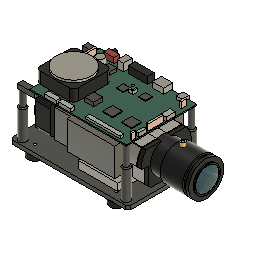
Projector v8 (Autodesk Fusion 360 design; units mm, degrees)
Autodesk Fusion 360 part; units mm, degrees
note: some values were not read from the file. Set by a fixed rule: which sketch regions a step uses.
sketch "Sketch1" plane through (0, 0, 0) normal (0, 0, 1) x (1, 0, 0)
  line L0 (0, 0) -> (155.5, 0)
  line L1 (155.5, 0) -> (155.5, 100)
  line L2 (155.5, 100) -> (0, 100)
  line L3 (0, 100) -> (0, 0)
  dimension "d1" = 155.5
  dimension "d2" = 100
  constraint horizontal L0
  constraint vertical L1
  constraint horizontal L2
  constraint vertical L3
  constraint coincident L0.start L3.end
  measures "d1" distance of L0.start L0.end
  measures "d2" distance of L0.start L2.end
extrude "Extrude1" add sketch "Sketch1" along normal blind 5 makes body 1
sketch "Sketch3" plane through (0, 0, 0) normal (0, 0, -1) x (1, 0, 0)
  line L0 (0, 0) -> (0, -100)
  line L1 (0, -100) -> (155.5, -100)
  line L2 (155.5, -100) -> (155.5, 0)
  line L3 (155.5, 0) -> (0, 0)
  line L4 (9.75, -7.15) -> (145.75, -7.15)
  line L5 (145.75, -7.15) -> (145.75, -92.85)
  line L6 (145.75, -92.85) -> (9.75, -92.85)
  line L7 (9.75, -92.85) -> (9.75, -7.15)
  line L8 (0, -50) -> (155.5, -50) construction
  line L9 (77.75, 0) -> (77.75, -100) construction
  line L10 (23, -9.75) -> (130.5, -9.75)
  line L11 (130.5, -9.75) -> (130.5, -90.25)
  line L12 (130.5, -90.25) -> (23, -90.25)
  line L13 (23, -90.25) -> (23, -9.75)
  dimension "d5" = 136
  dimension "d6" = 85.7
  dimension "d13" = 107.5
  dimension "d14" = 80.5
  dimension "d15" = 25
  dimension "d16" = 23
  constraint horizontal L4
  constraint vertical L5
  constraint horizontal L6
  constraint vertical L7
  constraint midpoint L0 L8.start
  constraint midpoint L2 L8.end
  constraint midpoint L3 L9.start
  constraint midpoint L1 L9.end
  constraint symmetric L4 L6 L8
  constraint symmetric L5 L7 L9
  constraint horizontal L10
  constraint vertical L11
  constraint horizontal L12
  constraint vertical L13
  constraint symmetric L8 L10 L12
  measures "d5" distance of L4.start L4.end
  measures "d6" distance of L4.start L6.end
  measures "d13" distance of L10.start L10.end
  measures "d14" distance of L10.end L11.end
  measures "d15" distance of L2 L11
  measures "d16" distance of L0 L13
hole "Hole1" at (9.75, 7.15, 0) at (145.75, 7.15, 0) at (145.75, 92.85, 0) at (9.75, 92.85, 0) direction (0, 0, 1) diameter 3 depth 5 tip angle 180 counterbore diameter 8 counterbore depth 3.5 bodies 1
chamfer "Chamfer1" distance 3.5 angle 45 4 edges at (0, 0, 2.5) (155.5, 0, 2.5) (0, 100, 2.5) (155.5, 100, 2.5) on bodies 1
hole "Hole2" at (23, 9.75, 0) at (130.5, 9.75, 0) at (130.5, 90.25, 0) at (23, 90.25, 0) direction (0, 0, 1) diameter 3.332 depth 5 tip angle 180 bodies 1
thread "Thread1" "ISO Metric profile 4.0 M4x0.7 6H"
sketch "Sketch4" plane through (0, 0, 0) normal (0, 0, 1) x (1, 0, 0) in component "Rubber Leg"
  circle A0 centre (0, 0) radius 10
  dimension "d20" = 20
  constraint coincident A0.centre origin
  measures "d20" diameter of A0
extrude "Extrude2" add sketch "Sketch4" along normal blind 8 separate body makes body 2 in component "Rubber Leg"
hole "Hole3" at (0, 0, 8) direction (0, 0, -1) diameter 4 depth 8 tip angle 180 counterbore diameter 8 counterbore depth 5 bodies 2 in component "Rubber Leg"
chamfer "Chamfer1'" distance 1 distance2 8 1 edges at (-9.3233, -3.6162, 8) measured on face at (7.959, -0.5964, 8) on bodies 2 in component "Rubber Leg"
pattern_linear "ఁ4" [suppressed]
sketch "Sketch2" plane through (0, 0, 0) normal (0, 0, 1) x (1, 0, 0) in component "Short Pole"
  circle A0 centre (0, 0) radius 5
  dimension "d38" = 10
  constraint coincident A0.centre origin
  measures "d38" diameter of A0
extrude "Extrude1'" add sketch "Sketch2" along normal blind 39 separate body makes body 3 in component "Short Pole"
sketch "Sketch3 (2)" plane through (0, 0, 39) normal (0, 0, 1) x (-1, 0, 0) in component "Short Pole"
  circle A0 centre (0, 0) radius 5
  circle A1 centre (0, 0) radius 3.5
  dimension "d41" = 7
  constraint coincident A0.centre A1.centre
  measures "d41" diameter of A1
extrude "Extrude2'" add sketch "Sketch3 (2)" along normal blind 19 contours A1 bodies 3 in component "Short Pole"
chamfer "Chamfer1''" distance 1.5 angle 45 1 edges at (-4.6616, -1.8081, 39) on bodies 3 in component "Short Pole"
sketch "Sketch2 (2)" plane through (0, 0, 0) normal (0, 0, 1) x (1, 0, 0) in component "Short Pole (1)"
  circle A0 centre (0, 0) radius 5
  dimension "d38_1" = 10
  constraint coincident A0.centre origin
  measures "d38_1" diameter of A0
extrude "Extrude1''" add sketch "Sketch2 (2)" along normal blind 39 separate body makes body 4 in component "Short Pole (1)"
sketch "Sketch3 (3)" plane through (0, 0, 39) normal (0, 0, 1) x (-1, 0, 0) in component "Short Pole (1)"
  circle A0 centre (0, 0) radius 5
  circle A1 centre (0, 0) radius 3.5
  dimension "d41_1" = 7
  constraint coincident A0.centre A1.centre
  measures "d41_1" diameter of A1
extrude "Extrude2''" add sketch "Sketch3 (3)" along normal blind 19 contours A1 bodies 4 in component "Short Pole (1)"
chamfer "Chamfer1'''" distance 1.5 angle 45 1 edges at (-4.6616, -1.8081, 39) on bodies 4 in component "Short Pole (1)"
sketch "Sketch2 (3)" plane through (0, 0, 0) normal (0, 0, 1) x (1, 0, 0) in component "Tall Pole"
  circle A0 centre (0, 0) radius 5
  dimension "d38_2" = 10
  constraint coincident A0.centre origin
  measures "d38_2" diameter of A0
extrude "Extrude1'''" add sketch "Sketch2 (3)" along normal blind 39 separate body makes body 5 in component "Tall Pole"
sketch "Sketch3 (4)" plane through (0, 0, 39) normal (0, 0, 1) x (-1, 0, 0) in component "Tall Pole"
  circle A0 centre (0, 0) radius 5
  circle A1 centre (0, 0) radius 3.5
  dimension "d41_2" = 7
  constraint coincident A0.centre A1.centre
  measures "d41_2" diameter of A1
extrude "Extrude2'''" add sketch "Sketch3 (4)" along normal blind 25 contours A1 bodies 5 in component "Tall Pole"
chamfer "Chamfer1''''" distance 1.5 angle 45 1 edges at (-4.6616, -1.8081, 39) on bodies 5 in component "Tall Pole"
sketch "Sketch2 (4)" plane through (0, 0, 0) normal (0, 0, 1) x (1, 0, 0) in component "Tall Pole (1)"
  circle A0 centre (0, 0) radius 5
  dimension "d38_1_1" = 10
  constraint coincident A0.centre origin
  measures "d38_1_1" diameter of A0
extrude "Extrude1''''" add sketch "Sketch2 (4)" along normal blind 39 separate body makes body 6 in component "Tall Pole (1)"
sketch "Sketch3 (5)" plane through (0, 0, 39) normal (0, 0, 1) x (-1, 0, 0) in component "Tall Pole (1)"
  circle A0 centre (0, 0) radius 5
  circle A1 centre (0, 0) radius 3.5
  dimension "d41_1_1" = 7
  constraint coincident A0.centre A1.centre
  measures "d41_1_1" diameter of A1
extrude "Extrude2''''" add sketch "Sketch3 (5)" along normal blind 25 contours A1 bodies 6 in component "Tall Pole (1)"
chamfer "Chamfer1'''''" distance 1.5 angle 45 1 edges at (-4.6616, -1.8081, 39) on bodies 6 in component "Tall Pole (1)"
sketch "Sketch6" plane through (-9.75, -7.15, 58) normal (0, 0, 1) x (-1, 0, 0) in component "Short Pole"
  circle A0 centre (-9.75, -7.15) radius 3.5
  line L0 (-6.25, -3.65) -> (-29.25, -3.65)
  line L1 (-29.25, -3.65) -> (-29.25, -10.65)
  line L2 (-29.25, -10.65) -> (-6.25, -10.65)
  line L3 (-6.25, -10.65) -> (-6.25, -3.65)
  dimension "d53" = 23
  dimension "d54" = 7
  constraint horizontal L0
  constraint vertical L1
  constraint horizontal L2
  constraint vertical L3
  constraint tangent A0 L2
  constraint tangent A0 L3
  measures "d53" distance of L0.start L0.end
  measures "d54" distance of L0.start L2.end
extrude "Extrude3" add sketch "Sketch6" along normal blind 6 separate body makes body 7 in component "Short Pole"
sketch "Sketch4 (2)" plane through (0, 0, 58) normal (0, 0, 1) x (-1, 0, 0) in component "Short Pole (1)"
  circle A0 centre (0, 0) radius 3.5
  line L0 (3.5, -3.5) -> (-19.5, -3.5)
  line L1 (-19.5, -3.5) -> (-19.5, 3.5)
  line L2 (-19.5, 3.5) -> (3.5, 3.5)
  line L3 (3.5, 3.5) -> (3.5, -3.5)
  dimension "d57" = 23
  dimension "d58" = 7
  constraint horizontal L0
  constraint vertical L1
  constraint horizontal L2
  constraint vertical L3
  constraint tangent A0 L0
  constraint tangent A0 L3
  measures "d57" distance of L0.start L0.end
  measures "d58" distance of L0.start L2.end
extrude "Extrude3'" add sketch "Sketch4 (2)" along normal blind 6 bodies 4 in component "Short Pole (1)"
ref_plane "WorkPlane1" through (77.75, 50, 69) normal (0, 0, 1) x (1, 0, 0)
sketch "Sketch7" plane through (77.75, 50, 69) normal (0, 0, 1) x (1, 0, 0)
  line L0 (-71.5, 39.35) -> (-48.5, 39.35)
  line L1 (-48.5, 39.35) -> (-48.5, 46.35)
  line L2 (-48.5, 46.35) -> (-71.5, 46.35)
  line L3 (-71.5, 46.35) -> (-71.5, 39.35)
  line L4 (-71.5, -39.35) -> (-71.5, -46.35)
  line L5 (-71.5, -46.35) -> (-48.5, -46.35)
  line L6 (-48.5, -46.35) -> (-48.5, -39.35)
  line L7 (-48.5, -39.35) -> (-71.5, -39.35)
  circle A0 centre (68, 42.85) radius 3.5
  circle A1 centre (68, -42.85) radius 3.5
  line L8 (-55.5, 46.35) -> (71.5, 46.35)
  line L9 (71.5, 46.35) -> (71.5, -46.35)
  line L10 (71.5, -46.35) -> (-55.5, -46.35)
  line L11 (-55.5, -46.35) -> (-55.5, 46.35)
  dimension "d62" = 7
  constraint horizontal L8
  constraint vertical L9
  constraint horizontal L10
  constraint vertical L11
  constraint tangent A0 L8
  constraint tangent A1 L10
  constraint tangent A1 L9
  measures "d62" distance of L1 L11
extrude "Extrude3''" add sketch "Sketch7" along normal blind 1.5 separate body contours L0 L1 L2 L8 L11 | L0 L1 L6 L7 A0 A1 L8 L9 L10 L11 | L5 L6 L7 L10 L11 | A0 L8 L9 | A0 | A1 | A1 L9 L10 makes body 8
ref_plane "WorkPlane2" through (85.75, 50, 79) normal (0, 0, 1) x (1, 0, 0)
sketch "Sketch9" plane through (85.75, 50, 79) normal (0, 0, 1) x (1, 0, 0)
  line L0 (-63.5, -46.35) -> (63.5, -46.35)
  line L1 (63.5, -46.35) -> (63.5, 46.35)
  line L2 (63.5, 46.35) -> (-63.5, 46.35)
  line L3 (-63.5, 46.35) -> (-63.5, -46.35)
  line L4 (-59.5, -42.35) -> (-9.5, -42.35)
  line L5 (-9.5, -42.35) -> (-9.5, 7.65)
  line L6 (-9.5, 7.65) -> (-59.5, 7.65)
  line L7 (-59.5, 7.65) -> (-59.5, -42.35)
  dimension "d68" = 50
  dimension "d69" = 50
  dimension "d70" = 4
  dimension "d71" = 4
  constraint horizontal L4
  constraint vertical L5
  constraint horizontal L6
  constraint vertical L7
  measures "d68" distance of L5.end L6.end
  measures "d69" distance of L4.end L5.end
  measures "d70" distance of L0 L4
  measures "d71" distance of L3 L7
extrude "Extrude4" add sketch "Sketch9" along normal blind 15 separate body contours L4 L5 L6 L7 makes body 9
fillet "Fillet1" radius 6 4 edges at (76.25, 7.65, 86.5) (76.25, 57.65, 86.5) (26.25, 7.65, 86.5) (26.25, 57.65, 86.5) on bodies 9
ref_plane "WorkPlane3" through (23, 50, 2.5) normal (-1, 0, 0) x (0, -1, 0)
sketch "Sketch10" plane through (23, 50, 2.5) normal (-1, 0, 0) x (0, 1, 0)
  line L0 (40, -58.5) -> (-40, -58.5)
  line L1 (-40, -58.5) -> (-40, -18.5)
  line L2 (-40, -18.5) -> (40, -18.5)
  line L3 (40, -18.5) -> (40, -58.5)
  line L4 (46.35, -66.5) -> (-46.35, -66.5)
  line L5 (-46.35, -66.5) -> (-46.35, -68)
  line L6 (-46.35, -68) -> (46.35, -68)
  line L7 (46.35, -68) -> (46.35, -66.5)
  line L8 (0, -66.5) -> (0, 0) construction
  dimension "d77" = 40
  dimension "d78" = 80
  dimension "d79" = 8
  constraint horizontal L0
  constraint vertical L1
  constraint horizontal L2
  constraint vertical L3
  constraint midpoint L4 L8.start
  constraint coincident L8.end origin
  constraint symmetric L1 L3 L8
  measures "d77" distance of L0.end L1.end
  measures "d78" distance of L0.start L0.end
  measures "d79" distance of L0 L4
extrude "Extrude5" add sketch "Sketch10" against normal blind 20 separate body contours L0 L1 L2 L3 makes body 10
fillet "Fillet2" radius 6 4 edges at (33, 90, 61) (33, 10, 61) (33, 90, 21) (33, 10, 21) on bodies 10
ref_plane "WorkPlane4" through (155.5, 50, 2.5) normal (1, 0, 0) x (0, 1, 0)
sketch "Sketch11" plane through (155.5, 50, 2.5) normal (1, 0, 0) x (0, 1, 0)
  line L0 (-46.35, 66.5) -> (46.35, 66.5)
  line L1 (46.35, 66.5) -> (46.35, 68)
  line L2 (46.35, 68) -> (-46.35, 68)
  line L3 (-46.35, 68) -> (-46.35, 66.5)
  line L4 (0, 66.5) -> (0, 0) construction
  circle A0 centre (0, 35.75) radius 20.75
  line L5 (-37, 55.5) -> (37, 55.5)
  line L6 (37, 55.5) -> (37, 9.5)
  line L7 (37, 9.5) -> (-37, 9.5)
  line L8 (-37, 9.5) -> (-37, 55.5)
  circle A1 centre (0, 35.75) radius 33
  line L9 (-37, 9.5) -> (-23, 9.5)
  line L10 (-23, 9.5) -> (-23, 35.75)
  line L11 (-23, 35.75) -> (-37, 35.75)
  line L12 (-37, 35.75) -> (-37, 9.5)
  line L13 (37, 9.5) -> (23, 9.5)
  line L14 (23, 9.5) -> (23, 35.75)
  line L15 (23, 35.75) -> (37, 35.75)
  line L16 (37, 35.75) -> (37, 9.5)
  dimension "d85" = 41.5
  dimension "d86" = 30.75
  dimension "d95" = 46
  dimension "d96" = 66
  dimension "d97" = 11
  dimension "d98" = 74
  dimension "d101" = 46
  constraint midpoint L0 L4.start
  constraint coincident L4.end origin
  constraint coincident L4 A0.centre
  constraint horizontal L5
  constraint vertical L6
  constraint horizontal L7
  constraint vertical L8
  constraint concentric A0 A1
  constraint symmetric L4 L6 L8
  constraint horizontal L9
  constraint vertical L10
  constraint horizontal L11
  constraint vertical L12
  constraint horizontal L13
  constraint vertical L14
  constraint horizontal L15
  constraint vertical L16
  constraint coincident A0.centre L15
  constraint coincident A0.centre L11
  constraint symmetric L4 L10 L14
  measures "d85" diameter of A0
  measures "d86" distance of L0 A0.centre
  measures "d95" distance of L5.end L6.end
  measures "d96" diameter of A1
  measures "d97" distance of L0 L5
  measures "d98" distance of L5.start L5.end
  measures "d101" distance of L10 L14
extrude "Extrude6" add sketch "Sketch11" along normal blind 15 separate body contours A0 L5 | A0 L5 makes body 11
sketch "Sketch12" plane through (170.5, 0, 0) normal (1, 0, 0) x (0, 1, 0)
  circle A0 centre (50, 38.25) radius 20.75
  circle A1 centre (50, 38.25) radius 23
  dimension "d89" = 46
  constraint concentric A0 A1
  measures "d89" diameter of A1
extrude "Extrude7" add sketch "Sketch12" along normal blind 37.5 contours A0 | A1 bodies 11
sketch "Sketch13" plane through (208, 0, 0) normal (1, 0, 0) x (0, 1, 0)
  circle A0 centre (50, 38.25) radius 23
  circle A1 centre (50, 38.25) radius 17.3
  dimension "d92" = 34.6
  constraint concentric A0 A1
  measures "d92" diameter of A1
extrude "Extrude8" add sketch "Sketch13" along normal blind 1.5 contours A1 bodies 11
extrude "Extrude9" add sketch "Sketch11" against normal blind 5 contours A0 L5 L7 A1 L10 L11 L14 L15 | A0 L5 | A0 L5 bodies 11
fillet "Fillet3" radius 1 6 edges at (153, 17, 38.25) (153, 27, 38.25) (153, 23.5626, 58) (153, 73, 38.25) (153, 83, 38.25) (153, 76.4374, 58) on bodies 11
ref_plane "WorkPlane5" through (149.5, 50, 36.0253) normal (-1, 0, 0) x (0, -1, 0)
sketch "Sketch14" plane through (149.5, 50, 36.0253) normal (-1, 0, 0) x (0, 1, 0)
  arc A0 (25.9314, -21.9747) -> (26.7418, -21.5606) centre (25.9314, -20.9747) ccw
  arc A1 (26.7418, -21.5606) -> (32.9839, -3.2559) centre (0, -2.2247) ccw
  arc A2 (32.9839, -3.2559) -> (31.9844, -2.2247) centre (31.9844, -3.2247) ccw
  line L0 (31.9844, -2.2247) -> (24, -2.2247)
  arc A3 (23, -1.2247) -> (24, -2.2247) centre (24, -1.2247) ccw
  line L1 (23, -1.2247) -> (23, 21.4396)
  arc A4 (23, 21.4396) -> (19.9984, 24.0253) centre (0, -2.2247) ccw
  line L2 (19.9984, 24.0253) -> (-19.9984, 24.0253)
  arc A5 (-19.9984, 24.0253) -> (-23, 21.4396) centre (0, -2.2247) ccw
  line L3 (-23, 21.4396) -> (-23, -1.2247)
  arc A6 (-24, -2.2247) -> (-23, -1.2247) centre (-24, -1.2247) ccw
  line L4 (-24, -2.2247) -> (-31.9844, -2.2247)
  arc A7 (-31.9844, -2.2247) -> (-32.9839, -3.2559) centre (-31.9844, -3.2247) ccw
  arc A8 (-32.9839, -3.2559) -> (-26.7418, -21.5606) centre (0, -2.2247) ccw
  arc A9 (-26.7418, -21.5606) -> (-25.9314, -21.9747) centre (-25.9314, -20.9747) ccw
  line L5 (-25.9314, -21.9747) -> (-6.364, -21.9747)
  arc A10 (-6.364, -21.9747) -> (6.364, -21.9747) centre (0, -2.2247) ccw
  line L6 (6.364, -21.9747) -> (25.9314, -21.9747)
  circle A11 centre (0, -2.2247) radius 20.75
extrude "Extrude10" add sketch "Sketch14" along normal blind 15 separate body makes body 12
extrude "Extrude11" add sketch "Sketch14" against normal blind 1 separate body contours A10 A11 makes body 13
combine "Combine1" operation add target body 13 tool bodies 11
ref_plane "WorkPlane6" through (77.75, 50, 7.5) normal (0, 0, 1) x (1, 0, 0)
sketch "Sketch15" plane through (77.75, 50, 7.5) normal (0, 0, 1) x (1, 0, 0)
  circle A0 centre (52.75, 40.25) radius 1.666
  circle A1 centre (-54.75, -40.25) radius 1.666
  circle A2 centre (52.75, -40.25) radius 1.666
  circle A3 centre (-54.75, 40.25) radius 1.666
  line L0 (77.75, 46.5) -> (74.25, 50)
  line L1 (74.25, 50) -> (-74.25, 50)
  line L2 (-74.25, 50) -> (-77.75, 46.5)
  line L3 (-77.75, 46.5) -> (-77.75, -46.5)
  line L4 (-77.75, -46.5) -> (-74.25, -50)
  line L5 (-74.25, -50) -> (74.25, -50)
  line L6 (74.25, -50) -> (77.75, -46.5)
  line L7 (77.75, -46.5) -> (77.75, 46.5)
  circle A4 centre (68, 42.85) radius 1.5
  circle A5 centre (-68, -42.85) radius 1.5
  circle A6 centre (68, -42.85) radius 1.5
  circle A7 centre (-68, 42.85) radius 1.5
  line L8 (56.75, -24) -> (56.75, -31.9844)
  line L9 (56.75, -31.9844) -> (56.75, -32.9844)
  line L10 (56.75, -26.7418) -> (56.75, -32.9839)
  line L11 (56.75, -25.9314) -> (56.75, -26.7418)
  line L12 (56.75, -25.9314) -> (56.75, -6.364)
  line L13 (56.75, 6.364) -> (56.75, -6.364)
  line L14 (56.75, 6.364) -> (56.75, 25.9314)
  line L15 (56.75, 26.7418) -> (56.75, 25.9314)
  line L16 (56.75, 32.9839) -> (56.75, 26.7418)
  line L17 (56.75, 32.9844) -> (56.75, 31.9844)
  line L18 (56.75, 31.9844) -> (56.75, 24)
  line L19 (56.75, 23) -> (56.75, 24)
  line L20 (56.75, 23) -> (56.75, 19.9984)
  line L21 (56.75, 19.9984) -> (56.75, -19.9984)
  line L22 (56.75, -19.9984) -> (56.75, -23)
  line L23 (56.75, -24) -> (56.75, -23)
  line L24 (3.75, -42) -> (55.75, -42)
  line L25 (55.75, -42) -> (55.75, 42)
  line L26 (55.75, 42) -> (3.75, 42)
  line L27 (3.75, 42) -> (3.75, -42)
  line L28 (-77.75, 0) -> (77.75, 0) construction
  dimension "d110" = 52
  dimension "d111" = 84
  dimension "d112" = 1
  constraint horizontal L24
  constraint vertical L25
  constraint horizontal L26
  constraint vertical L27
  constraint midpoint L3 L28.start
  constraint midpoint L7 L28.end
  constraint symmetric L24 L26 L28
  measures "d110" distance of L25.end L26.end
  measures "d111" distance of L24.start L26.end
  measures "d112" distance of L21 L25
extrude "Extrude12" add sketch "Sketch15" along normal blind 9.5 separate body contours A0 | A2 | L24 L25 L26 L27 makes body 14
ref_plane "WorkPlane7" through (77.75, 50, 23) normal (0, 0, 1) x (1, 0, 0)
sketch "Sketch16" plane through (77.75, 50, 23) normal (0, 0, 1) x (1, 0, 0)
  line L0 (-34.75, -34) -> (-34.75, -40)
  line L1 (-34.75, -34) -> (-34.75, 34)
  line L2 (-34.75, 40) -> (-34.75, 34)
  line L3 (-34.75, 40) -> (-34.75, 34)
  line L4 (-34.75, 34) -> (-34.75, -34)
  line L5 (-34.75, -34) -> (-34.75, -40)
  line L6 (3.75, 42) -> (3.75, -42)
  line L7 (3.75, -42) -> (55.75, -42)
  line L8 (55.75, -42) -> (55.75, 42)
  line L9 (55.75, 42) -> (3.75, 42)
  line L10 (-28.75, 40) -> (-7.75, 40)
  line L11 (-7.75, 40) -> (-7.75, -40)
  line L12 (-7.75, -40) -> (-28.75, -40)
  line L13 (-28.75, -40) -> (-28.75, 40)
  line L14 (-7.75, 45) -> (54.75, 45)
  line L15 (54.75, 45) -> (54.75, -45)
  line L16 (54.75, -45) -> (-7.75, -45)
  line L17 (-7.75, -45) -> (-7.75, 45)
  line L18 (55.75, 0) -> (3.75, 0) construction
  dimension "d116" = 6
  dimension "d117" = 1
  dimension "d118" = 21
  dimension "d119" = 90
  dimension "d120" = 80
  constraint horizontal L10
  constraint vertical L11
  constraint horizontal L12
  constraint vertical L13
  constraint horizontal L14
  constraint vertical L15
  constraint horizontal L16
  constraint vertical L17
  constraint midpoint L8 L18.start
  constraint midpoint L6 L18.end
  constraint symmetric L14 L16 L18
  constraint symmetric L10 L12 L18
  constraint collinear L11 L17
  measures "d116" distance of L1 L13
  measures "d117" distance of L8 L15
  measures "d118" distance of L10.start L10.end
  measures "d119" distance of L14 L16
  measures "d120" distance of L10 L12
extrude "Extrude13" add sketch "Sketch16" along normal blind 37 separate body contours L6 L7 L9 L15 | L6 L7 L9 L11 L14 L15 L16 L17 | L10 L11 L12 L13 L17 makes body 15
sketch "Sketch17" plane through (209.5, 0, 0) normal (1, 0, 0) x (0, 1, 0)
  circle A0 centre (50, 38.25) radius 17.3
  circle A1 centre (50, 38.25) radius 15.5
  dimension "d123" = 31
  constraint concentric A0 A1
  measures "d123" diameter of A1
extrude "Extrude14" cut sketch "Sketch17" against normal blind 0.5 contours A1 bodies 13
sketch "Sketch18" plane through (0, 0, 94) normal (0, 0, 1) x (-1, 0, 0)
  arc A0 (-32.25, -57.65) -> (-26.25, -51.65) centre (-32.25, -51.65) ccw
  line L0 (-26.25, -51.65) -> (-26.25, -13.65)
  arc A1 (-26.25, -13.65) -> (-32.25, -7.65) centre (-32.25, -13.65) ccw
  line L1 (-32.25, -7.65) -> (-70.25, -7.65)
  arc A2 (-70.25, -7.65) -> (-76.25, -13.65) centre (-70.25, -13.65) ccw
  line L2 (-76.25, -13.65) -> (-76.25, -51.65)
  arc A3 (-76.25, -51.65) -> (-70.25, -57.65) centre (-70.25, -51.65) ccw
  line L3 (-70.25, -57.65) -> (-32.25, -57.65)
  circle A4 centre (-51.25, -32.65) radius 23
  dimension "d126" = 46
  dimension "d127" = 25
  dimension "d128" = 25
  measures "d126" diameter of A4
  measures "d127" distance of L1 A4.centre
  measures "d128" distance of L0 A4.centre
extrude "Extrude15" add sketch "Sketch18" along normal blind 3 contours A4 bodies 9
sketch "Sketch19" plane through (23, 0, 0) normal (-1, 0, 0) x (0, -1, 0)
  arc A0 (-16, 21) -> (-10, 27) centre (-16, 27) ccw
  line L0 (-10, 27) -> (-10, 55)
  arc A1 (-10, 55) -> (-16, 61) centre (-16, 55) ccw
  line L1 (-16, 61) -> (-84, 61)
  arc A2 (-84, 61) -> (-90, 55) centre (-84, 55) ccw
  line L2 (-90, 55) -> (-90, 27)
  arc A3 (-90, 27) -> (-84, 21) centre (-84, 27) ccw
  line L3 (-84, 21) -> (-16, 21)
  line L4 (-90, 41) -> (-10, 41) construction
  line L5 (-50, 61) -> (-50, 21) construction
  circle A4 centre (-70, 41) radius 18
  circle A5 centre (-30, 41) radius 18
  dimension "d131" = 36
  dimension "d132" = 36
  dimension "d133" = 40
  constraint midpoint L2 L4.start
  constraint midpoint L0 L4.end
  constraint midpoint L1 L5.start
  constraint midpoint L3 L5.end
  constraint coincident L4 A4.centre
  constraint coincident L4 A5.centre
  constraint symmetric L5 A4.centre A5.centre
  measures "d131" diameter of A4
  measures "d132" diameter of A5
  measures "d133" distance of A4.centre A5.centre
extrude "Extrude16" add sketch "Sketch19" along normal blind 3 contours A4 | A5 bodies 10
sketch "Sketch20" plane through (0, 0, 70.5) normal (0, 0, 1) x (-1, 0, 0)
  line L0 (-22.25, -3.65) -> (-149.25, -3.65)
  line L1 (-149.25, -3.65) -> (-149.25, -96.35)
  line L2 (-149.25, -96.35) -> (-22.25, -96.35)
  line L3 (-22.25, -96.35) -> (-22.25, -3.65)
  line L4 (-69.25, -86.35) -> (-94.25, -86.35)
  line L5 (-94.25, -86.35) -> (-94.25, -95.35)
  line L6 (-94.25, -95.35) -> (-69.25, -95.35)
  line L7 (-69.25, -95.35) -> (-69.25, -86.35)
  line L8 (-101.25, -85.85) -> (-116.25, -85.85)
  line L9 (-116.25, -85.85) -> (-116.25, -97.85)
  line L10 (-116.25, -97.85) -> (-101.25, -97.85)
  line L11 (-101.25, -97.85) -> (-101.25, -85.85)
  line L12 (-130.25, -88.35) -> (-138.25, -88.35)
  line L13 (-138.25, -88.35) -> (-138.25, -97.35)
  line L14 (-138.25, -97.35) -> (-130.25, -97.35)
  line L15 (-130.25, -97.35) -> (-130.25, -88.35)
  line L16 (-56.25, -84.85) -> (-64.25, -84.85)
  line L17 (-64.25, -84.85) -> (-64.25, -96.35)
  line L18 (-64.25, -96.35) -> (-56.25, -96.35)
  line L19 (-56.25, -96.35) -> (-56.25, -84.85)
  line L20 (-35.25, -87.85) -> (-48.75, -87.85)
  line L21 (-48.75, -87.85) -> (-48.75, -95.35)
  line L22 (-48.75, -95.35) -> (-35.25, -95.35)
  line L23 (-35.25, -95.35) -> (-35.25, -87.85)
  line L24 (-96.25, -25.65) -> (-109.25, -25.65)
  line L25 (-109.25, -25.65) -> (-109.25, -38.65)
  line L26 (-109.25, -38.65) -> (-96.25, -38.65)
  line L27 (-96.25, -38.65) -> (-96.25, -25.65)
  line L28 (-121.25, -25.65) -> (-134.25, -25.65)
  line L29 (-134.25, -25.65) -> (-134.25, -38.65)
  line L30 (-134.25, -38.65) -> (-121.25, -38.65)
  line L31 (-121.25, -38.65) -> (-121.25, -25.65)
  line L32 (-141.75, -56.65) -> (-148.75, -56.65)
  line L33 (-148.75, -56.65) -> (-148.75, -68.65)
  line L34 (-148.75, -68.65) -> (-141.75, -68.65)
  line L35 (-141.75, -68.65) -> (-141.75, -56.65)
  circle A0 centre (-42.25, -76.35) radius 5
  line L36 (-90.25, -65.35) -> (-96.25, -65.35)
  line L37 (-96.25, -65.35) -> (-96.25, -71.35)
  line L38 (-96.25, -71.35) -> (-90.25, -71.35)
  line L39 (-90.25, -71.35) -> (-90.25, -65.35)
  line L40 (-145.25, -20.65) -> (-148.75, -20.65)
  line L41 (-148.75, -20.65) -> (-148.75, -30.65)
  line L42 (-148.75, -30.65) -> (-145.25, -30.65)
  line L43 (-145.25, -30.65) -> (-145.25, -20.65)
  line L44 (-103.25, -65.85) -> (-112.25, -65.85)
  line L45 (-112.25, -65.85) -> (-112.25, -74.85)
  line L46 (-112.25, -74.85) -> (-103.25, -74.85)
  line L47 (-103.25, -74.85) -> (-103.25, -65.85)
  line L48 (-49.25, -81.35) -> (-59.25, -81.35)
  line L49 (-59.25, -81.35) -> (-59.25, -71.35)
  line L50 (-59.25, -71.35) -> (-49.25, -71.35)
  line L51 (-49.25, -71.35) -> (-49.25, -81.35)
  line L52 (-84.25, -37.65) -> (-72.25, -37.65)
  line L53 (-72.25, -37.65) -> (-72.25, -25.65)
  line L54 (-72.25, -25.65) -> (-84.25, -25.65)
  line L55 (-84.25, -25.65) -> (-84.25, -37.65)
  line L56 (-138.25, -11.65) -> (-93.25, -11.65)
  line L57 (-93.25, -11.65) -> (-93.25, -6.65)
  line L58 (-93.25, -6.65) -> (-138.25, -6.65)
  line L59 (-138.25, -6.65) -> (-138.25, -11.65)
  line L60 (-147.75, -17.65) -> (-145.25, -17.65)
  line L61 (-145.25, -17.65) -> (-145.25, -12.65)
  line L62 (-145.25, -12.65) -> (-147.75, -12.65)
  line L63 (-147.75, -12.65) -> (-147.75, -17.65)
  line L64 (-145.25, -33.65) -> (-147.75, -33.65)
  line L65 (-147.75, -33.65) -> (-147.75, -53.65)
  line L66 (-147.75, -53.65) -> (-145.25, -53.65)
  line L67 (-145.25, -53.65) -> (-145.25, -33.65)
  line L68 (-26.75, -87.35) -> (-24.25, -87.35)
  line L69 (-24.25, -87.35) -> (-24.25, -67.35)
  line L70 (-24.25, -67.35) -> (-26.75, -67.35)
  line L71 (-26.75, -67.35) -> (-26.75, -87.35)
  line L72 (-87.75, -70.35) -> (-78.75, -70.35)
  line L73 (-78.75, -70.35) -> (-78.75, -61.35)
  line L74 (-78.75, -61.35) -> (-87.75, -61.35)
  line L75 (-87.75, -61.35) -> (-87.75, -70.35)
  line L76 (-144.25, -88.35) -> (-141.75, -88.35)
  line L77 (-141.75, -88.35) -> (-141.75, -80.85)
  line L78 (-141.75, -80.85) -> (-144.25, -80.85)
  line L79 (-144.25, -80.85) -> (-144.25, -88.35)
  line L80 (-75.75, -9.65) -> (-59.75, -9.65)
  line L81 (-59.75, -9.65) -> (-59.75, -3.65)
  line L82 (-59.75, -3.65) -> (-75.75, -3.65)
  line L83 (-75.75, -3.65) -> (-75.75, -9.65)
  line L84 (-57.25, -9.65) -> (-41.25, -9.65)
  line L85 (-41.25, -9.65) -> (-41.25, -3.65)
  line L86 (-41.25, -3.65) -> (-57.25, -3.65)
  line L87 (-57.25, -3.65) -> (-57.25, -9.65)
  line L88 (-22.25, -19.65) -> (-28.25, -19.65)
  line L89 (-28.25, -19.65) -> (-28.25, -35.65)
  line L90 (-28.25, -35.65) -> (-22.25, -35.65)
  line L91 (-22.25, -35.65) -> (-22.25, -19.65)
  dimension "d136" = 25
  dimension "d137" = 9
  dimension "d138" = 15
  dimension "d139" = 12
  dimension "d140" = 8
  dimension "d141" = 9
  dimension "d142" = 8
  dimension "d143" = 11.5
  dimension "d144" = 13.5
  dimension "d145" = 7.5
  dimension "d146" = 13
  dimension "d147" = 13
  dimension "d148" = 13
  dimension "d149" = 13
  dimension "d150" = 7
  dimension "d151" = 12
  dimension "d152" = 10
  dimension "d153" = 6
  dimension "d154" = 6
  dimension "d155" = 3.5
  dimension "d156" = 10
  dimension "d157" = 9
  dimension "d158" = 9
  dimension "d159" = 10
  dimension "d160" = 10
  dimension "d161" = 12
  dimension "d162" = 12
  dimension "d163" = 1
  dimension "d165" = 1
  dimension "d166" = 10.5
  dimension "d167" = 1
  dimension "d168" = 15
  dimension "d169" = 27
  dimension "d170" = 20
  dimension "d171" = 20
  dimension "d172" = 31
  dimension "d173" = 25
  dimension "d174" = 7
  dimension "d175" = 11
  dimension "d176" = 0.5
  dimension "d177" = 0.5
  dimension "d178" = 15
  dimension "d179" = 12
  dimension "d180" = 12
  dimension "d181" = 22
  dimension "d182" = 17
  dimension "d183" = 26
  dimension "d184" = 11
  dimension "d185" = 14
  dimension "d186" = 7
  dimension "d187" = 5
  dimension "d188" = 7.5
  dimension "d211" = 45
  dimension "d212" = 5
  dimension "d213" = 3
  dimension "d214" = 11
  dimension "d215" = 2.5
  dimension "d216" = 5
  dimension "d217" = 2.5
  dimension "d218" = 20
  dimension "d219" = 2.5
  dimension "d220" = 20
  dimension "d221" = 9
  dimension "d222" = 9
  dimension "d223" = 2.5
  dimension "d224" = 7.5
  dimension "d225" = 5
  dimension "d226" = 8
  dimension "d227" = 1.5
  dimension "d228" = 3
  dimension "d229" = 3
  dimension "d230" = 1.5
  dimension "d231" = 2
  dimension "d232" = 9
  dimension "d233" = 16
  dimension "d234" = 2.5
  dimension "d250" = 16
  dimension "d251" = 6
  dimension "d252" = 16
  dimension "d253" = 6
  dimension "d254" = 16
  dimension "d255" = 6
  dimension "d256" = 2.5
  dimension "d257" = 19
  dimension "d258" = 16
  constraint horizontal L4
  constraint vertical L5
  constraint horizontal L6
  constraint vertical L7
  constraint horizontal L8
  constraint vertical L9
  constraint horizontal L10
  constraint vertical L11
  constraint horizontal L12
  constraint vertical L13
  constraint horizontal L14
  constraint vertical L15
  constraint horizontal L16
  constraint vertical L17
  constraint horizontal L18
  constraint vertical L19
  constraint horizontal L20
  constraint vertical L21
  constraint horizontal L22
  constraint vertical L23
  constraint horizontal L24
  constraint vertical L25
  constraint horizontal L26
  constraint vertical L27
  constraint horizontal L28
  constraint vertical L29
  constraint horizontal L30
  constraint vertical L31
  constraint horizontal L32
  constraint vertical L33
  constraint horizontal L34
  constraint vertical L35
  constraint horizontal L36
  constraint vertical L37
  constraint horizontal L38
  constraint vertical L39
  constraint horizontal L40
  constraint vertical L41
  constraint horizontal L42
  constraint vertical L43
  constraint horizontal L44
  constraint vertical L45
  constraint horizontal L46
  constraint vertical L47
  constraint horizontal L48
  constraint vertical L49
  constraint horizontal L50
  constraint vertical L51
  constraint horizontal L52
  constraint vertical L53
  constraint horizontal L54
  constraint vertical L55
  constraint collinear L2 L18
  constraint collinear L26 L30
  constraint collinear L24 L54
  constraint horizontal L56
  constraint vertical L57
  constraint horizontal L58
  constraint vertical L59
  constraint horizontal L60
  constraint vertical L61
  constraint horizontal L62
  constraint vertical L63
  constraint horizontal L64
  constraint vertical L65
  constraint horizontal L66
  constraint vertical L67
  constraint horizontal L68
  constraint vertical L69
  constraint horizontal L70
  constraint vertical L71
  constraint horizontal L72
  constraint vertical L73
  constraint horizontal L74
  constraint vertical L75
  constraint horizontal L76
  constraint vertical L77
  constraint horizontal L78
  constraint vertical L79
  constraint horizontal L80
  constraint vertical L81
  constraint horizontal L82
  constraint vertical L83
  constraint horizontal L84
  constraint vertical L85
  constraint horizontal L86
  constraint vertical L87
  constraint horizontal L88
  constraint vertical L89
  constraint horizontal L90
  constraint vertical L91
  constraint collinear L3 L91
  constraint collinear L0 L86
  constraint collinear L0 L82
  measures "d136" distance of L4.start L4.end
  measures "d137" distance of L4.end L5.end
  measures "d138" distance of L8.start L8.end
  measures "d139" distance of L8.start L10.end
  measures "d140" distance of L12.start L12.end
  measures "d141" distance of L12.start L14.end
  measures "d142" distance of L16.start L16.end
  measures "d143" distance of L16.start L18.end
  measures "d144" distance of L20.start L20.end
  measures "d145" distance of L20.start L22.end
  measures "d146" distance of L24.start L24.end
  measures "d147" distance of L24.start L26.end
  measures "d148" distance of L28.start L28.end
  measures "d149" distance of L28.start L30.end
  measures "d150" distance of L32.start L32.end
  measures "d151" distance of L32.start L34.end
  measures "d152" diameter of A0
  measures "d153" distance of L36.start L36.end
  measures "d154" distance of L36.start L38.end
  measures "d155" distance of L40.start L40.end
  measures "d156" distance of L40.start L42.end
  measures "d157" distance of L44.start L44.end
  measures "d158" distance of L44.start L46.end
  measures "d159" distance of L48.start L48.end
  measures "d160" distance of L48.start L50.end
  measures "d161" distance of L52.start L52.end
  measures "d162" distance of L52.start L54.end
  measures "d163" distance of L2 L6
  measures "d165" distance of L2 L14
  measures "d166" distance of L2 L8
  measures "d167" distance of L2 L22
  measures "d168" distance of L2 L48
  measures "d169" distance of L3 L51
  measures "d170" distance of L3 A0.centre
  measures "d171" distance of L2 A0.centre
  measures "d172" distance of L39 L49
  measures "d173" distance of L2 L38
  measures "d174" distance of L37 L47
  measures "d175" distance of L8 L46
  measures "d176" distance of L1 L33
  measures "d177" distance of L1 L41
  measures "d178" distance of L1 L29
  measures "d179" distance of L25 L31
  measures "d180" distance of L27 L55
  measures "d181" distance of L0 L24
  measures "d182" distance of L0 L40
  measures "d183" distance of L32 L42
  measures "d184" distance of L1 L13
  measures "d185" distance of L9 L15
  measures "d186" distance of L5 L11
  measures "d187" distance of L7 L17
  measures "d188" distance of L19 L21
  measures "d211" distance of L56.start L56.end
  measures "d212" distance of L56.end L57.end
  measures "d213" distance of L0 L58
  measures "d214" distance of L1 L59
  measures "d215" distance of L60.start L60.end
  measures "d216" distance of L60.start L62.end
  measures "d217" distance of L64.start L64.end
  measures "d218" distance of L64.start L66.end
  measures "d219" distance of L68.start L68.end
  measures "d220" distance of L68.start L70.end
  measures "d221" distance of L72.start L72.end
  measures "d222" distance of L72.start L74.end
  measures "d223" distance of L76.start L76.end
  measures "d224" distance of L76.start L78.end
  measures "d225" distance of L1 L79
  measures "d226" distance of L2 L76
  measures "d227" distance of L1 L65
  measures "d228" distance of L42 L64
  measures "d229" distance of L40 L60
  measures "d230" distance of L1 L63
  measures "d231" distance of L3 L69
  measures "d232" distance of L2 L68
  measures "d233" distance of L4 L72
  measures "d234" distance of L39 L75
  measures "d250" distance of L80.start L80.end
  measures "d251" distance of L80.start L82.end
  measures "d252" distance of L84.start L84.end
  measures "d253" distance of L84.end L85.end
  measures "d254" distance of L88.end L89.end
  measures "d255" distance of L89.end L90.end
  measures "d256" distance of L81 L87
  measures "d257" distance of L3 L85
  measures "d258" distance of L0 L88
extrude "Extrude17" add sketch "Sketch20" along normal blind 1 separate body contours L24 L25 L26 L27 | L28 L29 L30 L31 | L44 L45 L46 L47 | L72 L73 L74 L75 makes body 16 at (104.9167, 29.9833, 70.5) makes body 17 at (109.25, 68.85, 70.5) makes body 18 at (129.9167, 29.9833, 70.5) makes body 19 at (84.75, 67.35, 70.5)
extrude "Extrude18" add sketch "Sketch20" along normal blind 5 separate body contours L52 L53 L54 L55 makes body 20
extrude "Extrude19" add sketch "Sketch20" along normal blind 4 separate body contours L48 L49 L50 L51 makes body 21
extrude "Extrude20" add sketch "Sketch20" along normal blind 11 separate body contours A0 makes body 22
extrude "Extrude21" add sketch "Sketch20" along normal blind 10 separate body contours L2 L16 L17 L18 L19 makes body 23
extrude "Extrude22" add sketch "Sketch20" along normal blind 9 separate body contours L4 L5 L6 L7 makes body 24
extrude "Extrude23" add sketch "Sketch20" along normal blind 7 separate body contours L2 L9 L10 L11 | L2 L8 L9 L11 makes body 25
extrude "Extrude24" add sketch "Sketch20" along normal blind 4 separate body contours L2 L12 L13 L15 | L2 L13 L14 L15 makes body 26
extrude "Extrude25" add sketch "Sketch20" along normal blind 5 separate body contours L32 L33 L34 L35 | L40 L41 L42 L43 makes body 27 at (146.4167, 60.65, 70.5) makes body 28 at (145.25, 27.3167, 72.1667)
extrude "Extrude26" add sketch "Sketch20" along normal blind 4 separate body contours L36 L37 L38 L39 makes body 29
extrude "Extrude27" add sketch "Sketch20" along normal blind 7 separate body contours L20 L21 L22 L23 makes body 30
extrude "Extrude28" add sketch "Sketch20" along normal blind 8 separate body contours L60 L61 L62 L63 | L64 L65 L66 L67 | L68 L69 L70 L71 | L76 L77 L78 L79 makes body 31 at (145.25, 15.9833, 73.1667) makes body 32 at (144.25, 83.35, 73.1667) makes body 33 at (145.25, 46.9833, 75.8333) makes body 34 at (26.75, 74.0167, 75.8333)
extrude "Extrude29" add sketch "Sketch20" along normal blind 3 separate body contours L56 L57 L58 L59 makes body 35
sketch "Sketch21" plane through (0, 0, 74.5) normal (0, 0, 1) x (-1, 0, 0)
  line L0 (-90.25, -71.35) -> (-90.25, -65.35)
  line L1 (-90.25, -65.35) -> (-96.25, -65.35)
  line L2 (-96.25, -65.35) -> (-96.25, -71.35)
  line L3 (-96.25, -71.35) -> (-90.25, -71.35)
  circle A0 centre (-93.25, -68.35) radius 1.75
  dimension "d239" = 3.5
  dimension "d248" = 3
  dimension "d249" = 3
  measures "d239" diameter of A0
  measures "d248" distance of L1 A0.centre
  measures "d249" distance of L2 A0.centre
extrude "Extrude30" add sketch "Sketch21" along normal blind 3.5 contours A0 bodies 29
sketch "Sketch22" plane through (0, 95.35, 0) normal (0, 1, 0) x (-1, 0, 0)
  line L0 (-48.75, 70.5) -> (-35.25, 70.5)
  line L1 (-35.25, 70.5) -> (-35.25, 77.5)
  line L2 (-35.25, 77.5) -> (-48.75, 77.5)
  line L3 (-48.75, 77.5) -> (-48.75, 70.5)
  line L4 (-41.25, 76) -> (-37.25, 76)
  line L5 (-37.25, 76) -> (-37.25, 72)
  line L6 (-37.25, 72) -> (-41.25, 72)
  line L7 (-41.25, 72) -> (-41.25, 76)
  dimension "d242" = 4
  dimension "d243" = 4
  dimension "d244" = 1.5
  dimension "d245" = 2
  constraint horizontal L4
  constraint vertical L5
  constraint horizontal L6
  constraint vertical L7
  measures "d242" distance of L4.start L4.end
  measures "d243" distance of L4.start L6.end
  measures "d244" distance of L2 L4
  measures "d245" distance of L1 L5
extrude "Extrude31" add sketch "Sketch22" along normal blind 5 contours L4 L5 L6 L7 bodies 30
extrude "Extrude32" add sketch "Sketch20" along normal blind 4.5 separate body contours L0 L84 L85 L86 L87 | L3 L88 L89 L90 L91 | L0 L80 L81 L82 L83 makes body 36 at (65.0833, 5.65, 70.5) makes body 37 at (46.5833, 5.65, 70.5) makes body 38 at (26.25, 24.9833, 70.5)
ref_plane "WorkPlane8" through (189.25, 50, 38.25) normal (0, -1, 0) x (1, 0, 0)
sketch "Sketch23" plane through (189.25, 50, 38.25) normal (0, -1, 0) x (1, 0, 0)
  line L0 (19.75, 15.5) -> (19.75, -15.5)
  circle A0 centre (-79.0414, 0) radius 100
  line L1 (19.75, 0) -> (20.9586, 0)
  dimension "d262" = 200
  constraint coincident L0.start A0
  constraint coincident L0.end A0
  constraint midpoint L0 L1.start
  constraint coincident A0 L1.end
  constraint perpendicular L0 L1
  measures "d262" diameter of A0
revolve "Revolve1" add sketch "Sketch23" angle 360 about axis through (151.75, 50, 38.25) along (1, 0, 0) separate body contours L0 A0 L1 picked at (20.5109, 1.7284) makes body 39
move_body "Move1" bodies 39 to x (1, 0, 0) y (0, 1, 0) z (0, 0, 1) at (0.01, 0, 0)
ref_plane "WorkPlane9" through (188.4953, 50, 61.25) normal (0, 0, 1) x (0, 1, 0)
sketch "Sketch24" plane through (188.4953, 50, 61.25) normal (0, 0, 1) x (1, 0, 0)
  line L0 (-17.9953, -23) -> (-17.9953, 23)
  line L1 (-17.9953, -20.75) -> (-17.9953, 20.75)
  line L2 (0, 0) -> (-17.9953, 0) construction
  circle A0 centre (-10.9953, 0) radius 3
  dimension "d265" = 6
  dimension "d266" = 7
  constraint coincident L2.start origin
  constraint midpoint L0 L2.end
  constraint coincident L2 A0.centre
  measures "d265" diameter of A0
  measures "d266" distance of L2.end A0.centre
extrude "Extrude33" add sketch "Sketch24" along normal blind 4.5 separate body makes body 40
move_face "OffsetFaces1" offset 1 1 faces at (178.2442, 50.5311, 61.25) on bodies 40
sketch "Sketch25" plane through (0, 0, 65.75) normal (0, 0, 1) x (-1, 0, 0)
  circle A0 centre (-177.5, -50) radius 3
  circle A1 centre (-177.5, -50) radius 1.75
  dimension "d270" = 3.5
  constraint concentric A0 A1
  measures "d270" diameter of A1
extrude "Extrude34" cut sketch "Sketch25" against normal blind 5 contours A1 bodies 40
ref_plane "WorkPlane10" through (204, 50, 38.25) normal (1, 0, 0) x (0, 1, 0)
sketch "Sketch26" plane through (204, 50, 38.25) normal (1, 0, 0) x (0, 1, 0)
  circle A0 centre (0, 0) radius 23
  circle A1 centre (0, 0) radius 23
  circle A2 centre (0, 0) radius 20.75
  dimension "d274" = 41.5
  constraint concentric A0 A2
  measures "d274" diameter of A2
extrude "Extrude35" cut sketch "Sketch26" against normal blind 4 bodies 13
component "Rubber Leg" placed x (1, 0, 0) y (0, -1, 0) z (0, 0, -1) at (23, 9.75, 0)
component "Rubber Leg" placed x (1, 0, 0) y (0, -1, 0) z (0, 0, -1) at (130.5, 9.75, 0)
component "Rubber Leg" placed x (1, 0, 0) y (0, -1, 0) z (0, 0, -1) at (23, 90.25, 0)
component "Rubber Leg" placed x (1, 0, 0) y (0, -1, 0) z (0, 0, -1) at (130.5, 90.25, 0)
component "Short Pole" placed x (1, 0, 0) y (0, 1, 0) z (0, 0, 1) at (9.75, 7.15, 5)
component "Short Pole (1)" placed x (1, 0, 0) y (0, 1, 0) z (0, 0, 1) at (9.75, 92.85, 5)
component "Tall Pole" placed x (1, 0, 0) y (0, 1, 0) z (0, 0, 1) at (145.75, 7.15, 5)
component "Tall Pole (1)" placed x (1, 0, 0) y (0, 1, 0) z (0, 0, 1) at (145.75, 92.85, 5)
equation "d86 = ( 41.5 / 2 ) * 1 mm + 10 mm"
equation "d111 = 100 mm - 16 mm"
named bodies: "Base", "PCB", "Top Fan", "Back Fans", "Lens Coupler", "Lens", "Bottom Heat Sink", "Main Heat Sink", "Chip1", "Chip2", "Chip3", "Chip4", "Pin1", "Pin2", "Pin3", "Pin4", "L1", "L2", "Cap", "Pwr", "2x7", "HDMI", "USB", "White1", "White2", "Btn", "Switch", "Bus", "LedR", "LedG", "LedB", "Glass"
